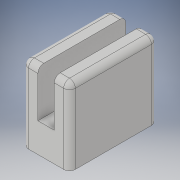
# Autodesk Inventor part: zoffset
Saved by Autodesk Inventor 2019 (Build 230136000, 136)
## iProperties
Created: 2019-10-25
Part Number: zoffset
Material: Generic
Document SubType Name: Modeling
Designer: assman
Density: 1 g/cm^3
Appearance: Default
Author: assman
## iProperties of the stored document zoffset_3DPrint.ipt
Created: 2019-10-25
Part Number: zoffset_3DPrint
Material: Generic
Document SubType Name: Modeling
Designer: assman
Density: 1 g/cm^3
Appearance: Default
Author: assman
Autodesk Inventor part; units mm, degrees
note: some values were not read from the file. Chosen so that the rebuilt part matches the saved one: direction of "Hole1".
ref_plane "YZ Plane" through (0, 0, 0) normal (1, 0, 0) x (0, 1, 0)
ref_plane "XZ Plane" through (0, 0, 0) normal (0, 1, 0) x (-1, 0, 0)
ref_plane "XY Plane" through (0, 0, 0) normal (0, 0, 1) x (1, 0, 0)
sketch "Sketch1" plane through (0, 0, 0) normal (0, 1, 0) x (-1, 0, 0)
  line L0 (4, 7.5) -> (-4, 7.5)
  line L1 (-4, 7.5) -> (-4, -7.5)
  line L2 (-4, -7.5) -> (4, -7.5)
  line L3 (4, -7.5) -> (4, 7.5)
  line L4 (4, 7.5) -> (-4, -7.5) construction
  line L5 (-4, 7.5) -> (4, -7.5) construction
  point P0 (0, 0)
  dimension "d0" = 8
  dimension "d1" = 15
  constraints: 12 end point, 2 midpoint, 2 parallel, 1 horizontal, 1 perpendicular
  measures "d0" distance of L2.end L1.end
  measures "d1" distance of L1.end L0.end
extrude "Extrusion1" add sketch "Sketch1" along normal blind 10
sketch "Sketch2" plane through (0, 10, 0) normal (0, 1, 0) x (1, 0, 0)
  line L0 (4, 7.5) -> (-4, 7.5) projected
  line L1 (-1.5, -7.5) -> (1.5, -7.5)
  line L2 (1.5, -7.5) -> (1.5, 7.5)
  line L3 (1.5, 7.5) -> (-1.5, 7.5)
  line L4 (-1.5, 7.5) -> (-1.5, -7.5)
  line L5 (-1.5, -7.5) -> (1.5, 7.5) construction
  line L6 (1.5, -7.5) -> (-1.5, 7.5) construction
  point P0 (0, 0)
  dimension "d4" = 3
  constraints: 12 end point, 2 midpoint, 2 parallel, 1 horizontal, 1 perpendicular, 1 point on line
  measures "d4" distance of L3.end L2.end
extrude "Extrusion2" cut sketch "Sketch2" against normal blind 5
thicken "Thicken1" operation add thickness 2 both sides no extend neighbours yes toward (0, 1, 0) faces at (2.3333, 10, -2.5)
thicken "Thicken2" operation add thickness 2 both sides no extend neighbours yes toward (0, 1, 0) faces at (-3.1667, 10, -2.5)
thicken "Thicken3" operation add thickness 1 both sides no extend neighbours yes toward (0, 1, 0) faces at (-3.1667, 12, -2.5)
thicken "Thicken4" operation add thickness 1 both sides no extend neighbours yes toward (0, 1, 0) faces at (3.1667, 12, 2.5)
fillet "Fillet1" radius 1 10 edges at (4, 6.5, 7.5) (4, 6.5, -7.5) (-4, 6.5, 7.5) (-4, 6.5, -7.5) (4, 13, 0) (-4, 13, 0) (2.75, 13, -7.5) (2.75, 13, 7.5) (-2.75, 13, 7.5) (-2.75, 13, -7.5)
sketch "Sketch3" plane through (0, 0, 0) normal (0, -1, 0) x (1, 0, 0)
  arc A0 (-3, 7.5) -> (-4, 6.5) centre (-3, 6.5) ccw construction
  line L0 (-4, -6.5) -> (-4, 6.5) construction
  arc A1 (-4, -6.5) -> (-3, -7.5) centre (-3, -6.5) ccw construction
  line L1 (3, -7.5) -> (-3, -7.5) construction
  arc A2 (3, -7.5) -> (4, -6.5) centre (3, -6.5) ccw construction
  line L2 (4, 6.5) -> (4, -6.5) construction
  arc A3 (4, 6.5) -> (3, 7.5) centre (3, 6.5) ccw construction
  line L3 (-3, 7.5) -> (3, 7.5) construction
  point P0 (0, 0)
  point P1 (0, 0)
  constraints: 1 coincident
hole "Hole1" at (0, 0, 0) direction (0, 1, 0) diameter 2.85 depth 5
thicken "Thicken7" operation add thickness 0.1 both sides no extend neighbours yes toward (-1, 0, 0) faces at (1.5, 7.6667, -2.1667)
thicken "Thicken8" operation add thickness 0.1 both sides no extend neighbours yes toward (1, 0, 0) faces at (-1.5, 7.6667, 2.1667)
body "Solid1"
